ESP32 Case (Autodesk Fusion 360 design; units mm, degrees)
Autodesk Fusion 360 part; units mm, degrees
sketch "ESP32 Base" plane through (0, 0, 0) normal (0, 1, 0) x (1, 0, 0)
  line L0 (0, 0) -> (28, 0)
  line L1 (28, 0) -> (28, 55)
  line L2 (28, 55) -> (0, 55)
  line L3 (0, 55) -> (0, 0)
  line L4 (-2, 57) -> (30, 57)
  line L5 (30, 57) -> (30, -2)
  line L6 (30, -2) -> (-2, -2)
  line L7 (-2, -2) -> (-2, 57)
  dimension "d1" = 28
  dimension "d2" = 55
  dimension "d3" = 2
  dimension "d4" = 2
  dimension "d5" = 2
  dimension "d6" = 2
  constraint horizontal L0
  constraint vertical L1
  constraint horizontal L2
  constraint vertical L3
  constraint coincident L0.start L3.end
  constraint horizontal L4
  constraint vertical L5
  constraint horizontal L6
  constraint vertical L7
  measures "d1" distance of L0.start L0.end
  measures "d2" distance of L0.start L2.end
  measures "d3" distance of L1 L5
  measures "d4" distance of L0 L6
  measures "d5" distance of L3 L7
  measures "d6" distance of L2 L4
sketch "ESP32 Front" plane through (0, 0, 0) normal (0, 0, 1) x (1, 0, 0)
  line L0 (0, 0) -> (28, 0)
  line L1 (28, 0) -> (28, 10)
  line L2 (28, 10) -> (0, 10)
  line L3 (0, 10) -> (0, 0)
  line L4 (9.5, 0) -> (18.5, 0)
  line L5 (18.5, 0) -> (18.5, 5)
  line L6 (18.5, 5) -> (9.5, 5)
  line L7 (9.5, 5) -> (9.5, 0)
  line L8 (-2, 12) -> (30, 12)
  line L9 (30, 12) -> (30, -2)
  line L10 (30, -2) -> (-2, -2)
  line L11 (-2, -2) -> (-2, 12)
  dimension "d7" = 28
  dimension "d8" = 10
  dimension "d9" = 9
  dimension "d10" = 5
  dimension "d11" = 9.5
  dimension "d12" = 2
  dimension "d13" = 2
  dimension "d14" = 2
  dimension "d15" = 2
  constraint horizontal L0
  constraint vertical L1
  constraint horizontal L2
  constraint vertical L3
  constraint coincident L0.start L3.end
  constraint horizontal L4
  constraint vertical L5
  constraint horizontal L6
  constraint vertical L7
  constraint coincident L0 L4.start
  constraint horizontal L8
  constraint vertical L9
  constraint horizontal L10
  constraint vertical L11
  measures "d7" distance of L0.start L0.end
  measures "d8" distance of L0.start L2.end
  measures "d9" distance of L4.start L4.end
  measures "d10" distance of L4.start L6.end
  measures "d11" distance of L3 L7
  measures "d12" distance of L2 L8
  measures "d13" distance of L1 L9
  measures "d14" distance of L3 L11
  measures "d15" distance of L0 L10
extrude "Extrude1" add sketch "ESP32 Base" along normal blind 2 from surface at -2 contours L0 L1 L2 L3 | L4 L5 L6 L7 makes body 1
extrude "Extrude2" add sketch "ESP32 Base" along normal blind 10 bodies 1
extrude "Extrude3" cut sketch "ESP32 Front" along normal blind 3 contours L0 L4 L5 L6 L7 bodies 1
sketch "ESP32 Lid" plane through (0, 0, 0) normal (0, 1, 0) x (1, 0, 0)
  line L0 (0, 0) -> (28, 0)
  line L1 (28, 0) -> (28, 55)
  line L2 (28, 55) -> (0, 55)
  line L3 (0, 55) -> (0, 0)
  line L4 (-2, 57) -> (30, 57)
  line L5 (30, 57) -> (30, -2)
  line L6 (30, -2) -> (-2, -2)
  line L7 (-2, -2) -> (-2, 57)
  line L8 (1.5, 53.5) -> (26.5, 53.5)
  line L9 (26.5, 53.5) -> (26.5, 1.5)
  line L10 (26.5, 1.5) -> (1.5, 1.5)
  line L11 (1.5, 1.5) -> (1.5, 53.5)
  dimension "d23" = 55
  dimension "d24" = 28
  dimension "d25" = 2
  dimension "d26" = 2
  dimension "d27" = 2
  dimension "d28" = 2
  dimension "d29" = 1.5
  dimension "d30" = 1.5
  dimension "d31" = 1.5
  dimension "d32" = 1.5
  constraint horizontal L0
  constraint vertical L1
  constraint horizontal L2
  constraint vertical L3
  constraint coincident L0.start L3.end
  constraint horizontal L4
  constraint vertical L5
  constraint horizontal L6
  constraint vertical L7
  constraint horizontal L8
  constraint vertical L9
  constraint horizontal L10
  constraint vertical L11
  measures "d23" distance of L0.start L2.end
  measures "d24" distance of L0.start L0.end
  measures "d25" distance of L2 L4
  measures "d26" distance of L1 L5
  measures "d27" distance of L0 L6
  measures "d28" distance of L3 L7
  measures "d29" distance of L2 L8
  measures "d30" distance of L1 L9
  measures "d31" distance of L3 L11
  measures "d32" distance of L0 L10
extrude "Extrude4" add sketch "ESP32 Lid" along normal blind 2 separate body contours L0 L1 L2 L3 | L4 L5 L6 L7 | L8 L9 L10 L11 makes body 2
extrude "Extrude5" add sketch "ESP32 Lid" along normal blind 5 contours L0 L1 L2 L3 bodies 2
fillet "Fillet1" radius 1.5 4 edges at (-2, 4, 2) (-2, 4, -57) (30, 4, 2) (30, 4, -57) on bodies 1
fillet "Fillet2" radius 1 4 edges at (18.5, 2.5, 2) (18.5, 2.5, 0) (9.5, 2.5, 0) (9.5, 2.5, 2) on bodies 1
fillet "Fillet3" radius 1.5 4 edges at (-2, 1, 2) (30, 1, 2) (30, 1, -57) (-2, 1, -57) on bodies 2
move_body "Move1" bodies 2 to x (1, 0, 0) y (0, 1, 0) z (0, 0, 1) at (45, 0, 0)
sketch "HomeAssistant" plane through (0, 0, 0) normal (0, 1, 0) x (1, 0, 0)
  spline S0 degree 3 poles (63.1801, 32.2819) (63.2605, 32.4605) (63.314, 32.6569) (63.314, 32.8623) knots 0 0 0 0 1 1 1 1
  spline S1 degree 3 poles (63.314, 32.8623) (63.314, 33.6035) (62.7157, 34.2018) (61.9746, 34.2018) knots 0 0 0 0 1 1 1 1
  spline S2 degree 3 poles (61.9746, 34.2018) (61.2334, 34.2018) (60.6351, 33.6035) (60.6351, 32.8623) knots 0 0 0 0 1 1 1 1
  spline S3 degree 3 poles (60.6351, 32.8623) (60.6351, 32.1211) (61.2334, 31.5229) (61.9746, 31.5229) knots 0 0 0 0 1 1 1 1
  spline S4 degree 3 poles (61.9746, 31.5229) (62.18, 31.5229) (62.3764, 31.5675) (62.555, 31.6568) knots 0 0 0 0 1 1 1 1
  line L0 (62.555, 31.6568) -> (64.4749, 29.728)
  line L1 (64.4749, 29.728) -> (64.4749, 27.8617)
  line L2 (64.4749, 27.8617) -> (62.0639, 25.4417)
  line L3 (62.0639, 25.4417) -> (62.0639, 27.2098)
  spline S5 degree 3 poles (62.0639, 27.2098) (62.5818, 27.3973) (62.9569, 27.8885) (62.9569, 28.4778) knots 0 0 0 0 1 1 1 1
  spline S6 degree 3 poles (62.9569, 28.4778) (62.9569, 29.219) (62.3586, 29.8173) (61.6174, 29.8173) knots 0 0 0 0 1 1 1 1
  spline S7 degree 3 poles (61.6174, 29.8173) (60.8762, 29.8173) (60.2779, 29.219) (60.2779, 28.4778) knots 0 0 0 0 1 1 1 1
  spline S8 degree 3 poles (60.2779, 28.4778) (60.2779, 27.8974) (60.653, 27.3973) (61.1709, 27.2098) knots 0 0 0 0 1 1 1 1
  line L4 (61.1709, 27.2098) -> (61.1709, 24.5398)
  line L5 (61.1709, 24.5398) -> (58.9385, 22.2985)
  line L6 (58.9385, 22.2985) -> (58.9385, 35.4519)
  line L7 (58.9385, 35.4519) -> (60.7691, 37.2914)
  spline S9 degree 3 poles (60.7691, 37.2914) (60.9477, 37.2111) (61.1352, 37.1575) (61.3495, 37.1575) knots 0 0 0 0 1 1 1 1
  spline S10 degree 3 poles (61.3495, 37.1575) (62.0907, 37.1575) (62.689, 37.7558) (62.689, 38.4969) knots 0 0 0 0 1 1 1 1
  spline S11 degree 3 poles (62.689, 38.4969) (62.689, 39.2381) (62.0907, 39.8364) (61.3495, 39.8364) knots 0 0 0 0 1 1 1 1
  spline S12 degree 3 poles (61.3495, 39.8364) (60.6083, 39.8364) (60.0101, 39.2381) (60.0101, 38.4969) knots 0 0 0 0 1 1 1 1
  spline S13 degree 3 poles (60.0101, 38.4969) (60.0101, 38.2916) (60.0547, 38.0951) (60.144, 37.9165) knots 0 0 0 0 1 1 1 1
  line L8 (60.144, 37.9165) -> (58.5009, 36.2645)
  line L9 (58.5009, 36.2645) -> (56.8579, 37.9165)
  spline S14 degree 3 poles (56.8579, 37.9165) (56.9382, 38.0951) (56.9918, 38.2916) (56.9918, 38.4969) knots 0 0 0 0 1 1 1 1
  spline S15 degree 3 poles (56.9918, 38.4969) (56.9918, 39.2381) (56.3935, 39.8364) (55.6524, 39.8364) knots 0 0 0 0 1 1 1 1
  spline S16 degree 3 poles (55.6524, 39.8364) (54.9112, 39.8364) (54.3129, 39.2381) (54.3129, 38.4969) knots 0 0 0 0 1 1 1 1
  spline S17 degree 3 poles (54.3129, 38.4969) (54.3129, 37.7558) (54.9112, 37.1575) (55.6524, 37.1575) knots 0 0 0 0 1 1 1 1
  spline S18 degree 3 poles (55.6524, 37.1575) (55.8577, 37.1575) (56.0542, 37.2021) (56.2328, 37.2914) knots 0 0 0 0 1 1 1 1
  line L10 (56.2328, 37.2914) -> (58.0634, 35.4519)
  line L11 (58.0634, 35.4519) -> (58.0634, 26.0579)
  line L12 (58.0634, 26.0579) -> (54.8487, 29.2815)
  line L13 (54.8487, 29.2815) -> (54.8487, 31.8622)
  spline S19 degree 3 poles (54.8487, 31.8622) (55.3666, 32.0497) (55.7417, 32.5408) (55.7417, 33.1302) knots 0 0 0 0 1 1 1 1
  spline S20 degree 3 poles (55.7417, 33.1302) (55.7417, 33.8714) (55.1434, 34.4696) (54.4022, 34.4696) knots 0 0 0 0 1 1 1 1
  spline S21 degree 3 poles (54.4022, 34.4696) (53.661, 34.4696) (53.0628, 33.8714) (53.0628, 33.1302) knots 0 0 0 0 1 1 1 1
  spline S22 degree 3 poles (53.0628, 33.1302) (53.0628, 32.5498) (53.4378, 32.0497) (53.9557, 31.8622) knots 0 0 0 0 1 1 1 1
  line L14 (53.9557, 31.8622) -> (53.9557, 30.1834)
  line L15 (53.9557, 30.1834) -> (51.4554, 32.6926)
  line L16 (51.4554, 32.6926) -> (51.4554, 35.184)
  spline S23 degree 3 poles (51.4554, 35.184) (51.9733, 35.3715) (52.3484, 35.8627) (52.3484, 36.452) knots 0 0 0 0 1 1 1 1
  spline S24 degree 3 poles (52.3484, 36.452) (52.3484, 37.1932) (51.7501, 37.7915) (51.0089, 37.7915) knots 0 0 0 0 1 1 1 1
  spline S25 degree 3 poles (51.0089, 37.7915) (50.2678, 37.7915) (49.6695, 37.1932) (49.6695, 36.452) knots 0 0 0 0 1 1 1 1
  spline S26 degree 3 poles (49.6695, 36.452) (49.6695, 35.8716) (50.0445, 35.3715) (50.5624, 35.184) knots 0 0 0 0 1 1 1 1
  line L17 (50.5624, 35.184) -> (50.5624, 32.3265)
  line L18 (50.5624, 32.3265) -> (53.3217, 29.5583)
  line L19 (53.3217, 29.5583) -> (51.7233, 29.5583)
  spline S27 degree 3 poles (51.7233, 29.5583) (51.5358, 30.0762) (51.0446, 30.4513) (50.4642, 30.4513) knots 0 0 0 0 1 1 1 1
  spline S28 degree 3 poles (50.4642, 30.4513) (49.7231, 30.4513) (49.1248, 29.853) (49.1248, 29.1118) knots 0 0 0 0 1 1 1 1
  spline S29 degree 3 poles (49.1248, 29.1118) (49.1248, 28.3707) (49.7231, 27.7724) (50.4642, 27.7724) knots 0 0 0 0 1 1 1 1
  spline S30 degree 3 poles (50.4642, 27.7724) (51.0446, 27.7724) (51.5447, 28.1474) (51.7233, 28.6654) knots 0 0 0 0 1 1 1 1
  line L20 (51.7233, 28.6654) -> (54.2058, 28.6654)
  line L21 (54.2058, 28.6654) -> (58.0455, 24.8077)
  line L22 (58.0455, 24.8077) -> (58.0455, 18.1015)
  line L23 (58.0455, 18.1015) -> (55.9917, 20.1643)
  line L24 (55.9917, 20.1643) -> (55.9917, 22.745)
  spline S31 degree 3 poles (55.9917, 22.745) (56.5096, 22.9325) (56.8847, 23.4236) (56.8847, 24.013) knots 0 0 0 0 1 1 1 1
  spline S32 degree 3 poles (56.8847, 24.013) (56.8847, 24.7541) (56.2864, 25.3524) (55.5452, 25.3524) knots 0 0 0 0 1 1 1 1
  spline S33 degree 3 poles (55.5452, 25.3524) (54.804, 25.3524) (54.2058, 24.7541) (54.2058, 24.013) knots 0 0 0 0 1 1 1 1
  spline S34 degree 3 poles (54.2058, 24.013) (54.2058, 23.4326) (54.5808, 22.9325) (55.0987, 22.745) knots 0 0 0 0 1 1 1 1
  line L25 (55.0987, 22.745) -> (55.0987, 21.0662)
  line L26 (55.0987, 21.0662) -> (52.1162, 24.0666)
  spline S35 degree 3 poles (52.1162, 24.0666) (52.1966, 24.2452) (52.2502, 24.4416) (52.2502, 24.647) knots 0 0 0 0 1 1 1 1
  spline S36 degree 3 poles (52.2502, 24.647) (52.2502, 25.3882) (51.6519, 25.9864) (50.9107, 25.9864) knots 0 0 0 0 1 1 1 1
  spline S37 degree 3 poles (50.9107, 25.9864) (50.1695, 25.9864) (49.5712, 25.3882) (49.5712, 24.647) knots 0 0 0 0 1 1 1 1
  spline S38 degree 3 poles (49.5712, 24.647) (49.5712, 23.9058) (50.1695, 23.3075) (50.9107, 23.3075) knots 0 0 0 0 1 1 1 1
  spline S39 degree 3 poles (50.9107, 23.3075) (51.1161, 23.3075) (51.3125, 23.3522) (51.4911, 23.4415) knots 0 0 0 0 1 1 1 1
  line L27 (51.4911, 23.4415) -> (54.4736, 20.4411)
  line L28 (54.4736, 20.4411) -> (52.8842, 20.4411)
  spline S40 degree 3 poles (52.8842, 20.4411) (52.6966, 20.959) (52.2055, 21.3341) (51.6251, 21.3341) knots 0 0 0 0 1 1 1 1
  spline S41 degree 3 poles (51.6251, 21.3341) (50.8839, 21.3341) (50.2856, 20.7358) (50.2856, 19.9946) knots 0 0 0 0 1 1 1 1
  spline S42 degree 3 poles (50.2856, 19.9946) (50.2856, 19.2535) (50.8839, 18.6552) (51.6251, 18.6552) knots 0 0 0 0 1 1 1 1
  spline S43 degree 3 poles (51.6251, 18.6552) (52.2055, 18.6552) (52.7056, 19.0302) (52.8842, 19.5481) knots 0 0 0 0 1 1 1 1
  line L29 (52.8842, 19.5481) -> (55.3666, 19.5481)
  line L30 (55.3666, 19.5481) -> (57.8669, 17.0389)
  line L31 (57.8669, 17.0389) -> (59.126, 17.0389)
  line L32 (59.126, 17.0389) -> (61.7156, 19.6374)
  line L33 (61.7156, 19.6374) -> (64.1088, 19.6374)
  spline S44 degree 3 poles (64.1088, 19.6374) (64.2963, 19.1195) (64.7874, 18.7445) (65.3679, 18.7445) knots 0 0 0 0 1 1 1 1
  spline S45 degree 3 poles (65.3679, 18.7445) (66.109, 18.7445) (66.7073, 19.3428) (66.7073, 20.0839) knots 0 0 0 0 1 1 1 1
  spline S46 degree 3 poles (66.7073, 20.0839) (66.7073, 20.8251) (66.109, 21.4234) (65.3679, 21.4234) knots 0 0 0 0 1 1 1 1
  spline S47 degree 3 poles (65.3679, 21.4234) (64.7874, 21.4234) (64.2874, 21.0483) (64.1088, 20.5304) knots 0 0 0 0 1 1 1 1
  line L34 (64.1088, 20.5304) -> (61.3495, 20.5304)
  line L35 (61.3495, 20.5304) -> (58.9474, 18.1194)
  line L36 (58.9474, 18.1194) -> (58.9474, 21.0662)
  line L37 (58.9474, 21.0662) -> (61.8049, 23.9415)
  line L38 (61.8049, 23.9415) -> (66.4216, 23.9415)
  spline S48 degree 3 poles (66.4216, 23.9415) (66.6091, 23.4236) (67.1002, 23.0486) (67.6807, 23.0486) knots 0 0 0 0 1 1 1 1
  spline S49 degree 3 poles (67.6807, 23.0486) (68.4218, 23.0486) (69.0201, 23.6469) (69.0201, 24.388) knots 0 0 0 0 1 1 1 1
  spline S50 degree 3 poles (69.0201, 24.388) (69.0201, 25.1292) (68.4218, 25.7275) (67.6807, 25.7275) knots 0 0 0 0 1 1 1 1
  spline S51 degree 3 poles (67.6807, 25.7275) (67.1002, 25.7275) (66.6002, 25.3524) (66.4216, 24.8345) knots 0 0 0 0 1 1 1 1
  line L39 (66.4216, 24.8345) -> (62.6979, 24.8345)
  line L40 (62.6979, 24.8345) -> (65.3679, 27.5134)
  line L41 (65.3679, 27.5134) -> (65.3679, 29.7548)
  line L42 (65.3679, 29.7548) -> (67.2877, 31.6836)
  spline S52 degree 3 poles (67.2877, 31.6836) (67.4663, 31.6032) (67.6539, 31.5496) (67.8682, 31.5496) knots 0 0 0 0 1 1 1 1
  spline S53 degree 3 poles (67.8682, 31.5496) (68.6093, 31.5496) (69.2076, 32.1479) (69.2076, 32.8891) knots 0 0 0 0 1 1 1 1
  spline S54 degree 3 poles (69.2076, 32.8891) (69.2076, 33.6303) (68.6093, 34.2285) (67.8682, 34.2285) knots 0 0 0 0 1 1 1 1
  spline S55 degree 3 poles (67.8682, 34.2285) (67.127, 34.2285) (66.5287, 33.6303) (66.5287, 32.8891) knots 0 0 0 0 1 1 1 1
  spline S56 degree 3 poles (66.5287, 32.8891) (66.5287, 32.6837) (66.5734, 32.4873) (66.6627, 32.3087) knots 0 0 0 0 1 1 1 1
  line L43 (66.6627, 32.3087) -> (65.3679, 31.0139)
  line L44 (65.3679, 31.0139) -> (65.3679, 35.1126)
  spline S57 degree 3 poles (65.3679, 35.1126) (65.8858, 35.3001) (66.2608, 35.7912) (66.2608, 36.3806) knots 0 0 0 0 1 1 1 1
  spline S58 degree 3 poles (66.2608, 36.3806) (66.2608, 37.1218) (65.6625, 37.7201) (64.9214, 37.7201) knots 0 0 0 0 1 1 1 1
  spline S59 degree 3 poles (64.9214, 37.7201) (64.1802, 37.7201) (63.5819, 37.1218) (63.5819, 36.3806) knots 0 0 0 0 1 1 1 1
  spline S60 degree 3 poles (63.5819, 36.3806) (63.5819, 35.8002) (63.957, 35.3001) (64.4749, 35.1126) knots 0 0 0 0 1 1 1 1
  line L45 (64.4749, 35.1126) -> (64.4749, 31.0139)
  line L46 (64.4749, 31.0139) -> (63.1801, 32.2819)
sketch "Sketch6" plane through (0, 0, 0) normal (0, 1, 0) x (1, 0, 0)
  line L0 (36.9451, 52.3701) -> (79.5148, 52.3701)
  line L1 (79.5148, 52.3701) -> (79.5148, 14.6379)
  line L2 (79.5148, 14.6379) -> (36.9451, 14.6379)
  line L3 (36.9451, 14.6379) -> (36.9451, 52.3701)
  spline S0 degree 3 poles (63.8629, 33.0203) (63.9596, 33.2353) (64.0241, 33.4718) (64.0241, 33.719) knots 0 0 0 0 1 1 1 1
  spline S1 degree 3 poles (64.0241, 33.719) (64.0241, 34.6113) (63.3039, 35.3315) (62.4116, 35.3315) knots 0 0 0 0 1 1 1 1
  spline S2 degree 3 poles (62.4116, 35.3315) (61.5194, 35.3315) (60.7992, 34.6113) (60.7992, 33.719) knots 0 0 0 0 1 1 1 1
  spline S3 degree 3 poles (60.7992, 33.719) (60.7992, 32.8268) (61.5194, 32.1065) (62.4116, 32.1065) knots 0 0 0 0 1 1 1 1
  spline S4 degree 3 poles (62.4116, 32.1065) (62.6589, 32.1065) (62.8954, 32.1603) (63.1104, 32.2678) knots 0 0 0 0 1 1 1 1
  line L4 (63.1104, 32.2678) -> (65.4216, 29.9458)
  line L5 (65.4216, 29.9458) -> (65.4216, 27.6991)
  line L6 (65.4216, 27.6991) -> (62.5191, 24.7859)
  line L7 (62.5191, 24.7859) -> (62.5191, 26.9143)
  spline S5 degree 3 poles (62.5191, 26.9143) (63.1426, 27.1401) (63.5941, 27.7313) (63.5941, 28.4408) knots 0 0 0 0 1 1 1 1
  spline S6 degree 3 poles (63.5941, 28.4408) (63.5941, 29.3331) (62.8739, 30.0533) (61.9816, 30.0533) knots 0 0 0 0 1 1 1 1
  spline S7 degree 3 poles (61.9816, 30.0533) (61.0894, 30.0533) (60.3692, 29.3331) (60.3692, 28.4408) knots 0 0 0 0 1 1 1 1
  spline S8 degree 3 poles (60.3692, 28.4408) (60.3692, 27.7421) (60.8207, 27.1401) (61.4442, 26.9143) knots 0 0 0 0 1 1 1 1
  line L8 (61.4442, 26.9143) -> (61.4442, 23.7001)
  line L9 (61.4442, 23.7001) -> (58.7567, 21.0019)
  line L10 (58.7567, 21.0019) -> (58.7567, 36.8365)
  line L11 (58.7567, 36.8365) -> (60.9604, 39.051)
  spline S9 degree 3 poles (60.9604, 39.051) (61.1754, 38.9542) (61.4012, 38.8897) (61.6592, 38.8897) knots 0 0 0 0 1 1 1 1
  spline S10 degree 3 poles (61.6592, 38.8897) (62.5514, 38.8897) (63.2716, 39.61) (63.2716, 40.5022) knots 0 0 0 0 1 1 1 1
  spline S11 degree 3 poles (63.2716, 40.5022) (63.2716, 41.3945) (62.5514, 42.1147) (61.6592, 42.1147) knots 0 0 0 0 1 1 1 1
  spline S12 degree 3 poles (61.6592, 42.1147) (60.7669, 42.1147) (60.0467, 41.3945) (60.0467, 40.5022) knots 0 0 0 0 1 1 1 1
  spline S13 degree 3 poles (60.0467, 40.5022) (60.0467, 40.255) (60.1004, 40.0185) (60.2079, 39.8035) knots 0 0 0 0 1 1 1 1
  line L12 (60.2079, 39.8035) -> (58.2299, 37.8148)
  line L13 (58.2299, 37.8148) -> (56.2519, 39.8035)
  spline S14 degree 3 poles (56.2519, 39.8035) (56.3487, 40.0185) (56.4132, 40.255) (56.4132, 40.5022) knots 0 0 0 0 1 1 1 1
  spline S15 degree 3 poles (56.4132, 40.5022) (56.4132, 41.3945) (55.6929, 42.1147) (54.8007, 42.1147) knots 0 0 0 0 1 1 1 1
  spline S16 degree 3 poles (54.8007, 42.1147) (53.9085, 42.1147) (53.1882, 41.3945) (53.1882, 40.5022) knots 0 0 0 0 1 1 1 1
  spline S17 degree 3 poles (53.1882, 40.5022) (53.1882, 39.61) (53.9085, 38.8897) (54.8007, 38.8897) knots 0 0 0 0 1 1 1 1
  spline S18 degree 3 poles (54.8007, 38.8897) (55.048, 38.8897) (55.2845, 38.9435) (55.4995, 39.051) knots 0 0 0 0 1 1 1 1
  line L14 (55.4995, 39.051) -> (57.7032, 36.8365)
  line L15 (57.7032, 36.8365) -> (57.7032, 25.5276)
  line L16 (57.7032, 25.5276) -> (53.8332, 29.4083)
  line L17 (53.8332, 29.4083) -> (53.8332, 32.515)
  spline S19 degree 3 poles (53.8332, 32.515) (54.4567, 32.7408) (54.9082, 33.332) (54.9082, 34.0415) knots 0 0 0 0 1 1 1 1
  spline S20 degree 3 poles (54.9082, 34.0415) (54.9082, 34.9338) (54.188, 35.654) (53.2957, 35.654) knots 0 0 0 0 1 1 1 1
  spline S21 degree 3 poles (53.2957, 35.654) (52.4035, 35.654) (51.6832, 34.9338) (51.6832, 34.0415) knots 0 0 0 0 1 1 1 1
  spline S22 degree 3 poles (51.6832, 34.0415) (51.6832, 33.3428) (52.1347, 32.7408) (52.7582, 32.515) knots 0 0 0 0 1 1 1 1
  line L18 (52.7582, 32.515) -> (52.7582, 30.4941)
  line L19 (52.7582, 30.4941) -> (49.7482, 33.5148)
  line L20 (49.7482, 33.5148) -> (49.7482, 36.514)
  spline S23 degree 3 poles (49.7482, 36.514) (50.3717, 36.7398) (50.8232, 37.331) (50.8232, 38.0405) knots 0 0 0 0 1 1 1 1
  spline S24 degree 3 poles (50.8232, 38.0405) (50.8232, 38.9327) (50.103, 39.653) (49.2107, 39.653) knots 0 0 0 0 1 1 1 1
  spline S25 degree 3 poles (49.2107, 39.653) (48.3185, 39.653) (47.5983, 38.9327) (47.5983, 38.0405) knots 0 0 0 0 1 1 1 1
  spline S26 degree 3 poles (47.5983, 38.0405) (47.5983, 37.3418) (48.0498, 36.7398) (48.6733, 36.514) knots 0 0 0 0 1 1 1 1
  line L21 (48.6733, 36.514) -> (48.6733, 33.074)
  line L22 (48.6733, 33.074) -> (51.995, 29.7416)
  line L23 (51.995, 29.7416) -> (50.0707, 29.7416)
  spline S27 degree 3 poles (50.0707, 29.7416) (49.845, 30.3651) (49.2537, 30.8166) (48.555, 30.8166) knots 0 0 0 0 1 1 1 1
  spline S28 degree 3 poles (48.555, 30.8166) (47.6628, 30.8166) (46.9425, 30.0963) (46.9425, 29.2041) knots 0 0 0 0 1 1 1 1
  spline S29 degree 3 poles (46.9425, 29.2041) (46.9425, 28.3118) (47.6628, 27.5916) (48.555, 27.5916) knots 0 0 0 0 1 1 1 1
  spline S30 degree 3 poles (48.555, 27.5916) (49.2537, 27.5916) (49.8557, 28.0431) (50.0707, 28.6666) knots 0 0 0 0 1 1 1 1
  line L24 (50.0707, 28.6666) -> (53.0592, 28.6666)
  line L25 (53.0592, 28.6666) -> (57.6817, 24.0226)
  line L26 (57.6817, 24.0226) -> (57.6817, 15.9494)
  line L27 (57.6817, 15.9494) -> (55.2092, 18.4327)
  line L28 (55.2092, 18.4327) -> (55.2092, 21.5394)
  spline S31 degree 3 poles (55.2092, 21.5394) (55.8327, 21.7651) (56.2842, 22.3564) (56.2842, 23.0659) knots 0 0 0 0 1 1 1 1
  spline S32 degree 3 poles (56.2842, 23.0659) (56.2842, 23.9581) (55.5639, 24.6784) (54.6717, 24.6784) knots 0 0 0 0 1 1 1 1
  spline S33 degree 3 poles (54.6717, 24.6784) (53.7795, 24.6784) (53.0592, 23.9581) (53.0592, 23.0659) knots 0 0 0 0 1 1 1 1
  spline S34 degree 3 poles (53.0592, 23.0659) (53.0592, 22.3671) (53.5107, 21.7651) (54.1342, 21.5394) knots 0 0 0 0 1 1 1 1
  line L29 (54.1342, 21.5394) -> (54.1342, 19.5184)
  line L30 (54.1342, 19.5184) -> (50.5437, 23.1304)
  spline S35 degree 3 poles (50.5437, 23.1304) (50.6405, 23.3454) (50.705, 23.5819) (50.705, 23.8291) knots 0 0 0 0 1 1 1 1
  spline S36 degree 3 poles (50.705, 23.8291) (50.705, 24.7214) (49.9847, 25.4416) (49.0925, 25.4416) knots 0 0 0 0 1 1 1 1
  spline S37 degree 3 poles (49.0925, 25.4416) (48.2003, 25.4416) (47.48, 24.7214) (47.48, 23.8291) knots 0 0 0 0 1 1 1 1
  spline S38 degree 3 poles (47.48, 23.8291) (47.48, 22.9369) (48.2003, 22.2166) (49.0925, 22.2166) knots 0 0 0 0 1 1 1 1
  spline S39 degree 3 poles (49.0925, 22.2166) (49.3397, 22.2166) (49.5762, 22.2704) (49.7912, 22.3779) knots 0 0 0 0 1 1 1 1
  line L31 (49.7912, 22.3779) -> (53.3817, 18.7659)
  line L32 (53.3817, 18.7659) -> (51.4682, 18.7659)
  spline S40 degree 3 poles (51.4682, 18.7659) (51.2425, 19.3894) (50.6512, 19.8409) (49.9525, 19.8409) knots 0 0 0 0 1 1 1 1
  spline S41 degree 3 poles (49.9525, 19.8409) (49.0603, 19.8409) (48.34, 19.1207) (48.34, 18.2284) knots 0 0 0 0 1 1 1 1
  spline S42 degree 3 poles (48.34, 18.2284) (48.34, 17.3362) (49.0603, 16.6159) (49.9525, 16.6159) knots 0 0 0 0 1 1 1 1
  spline S43 degree 3 poles (49.9525, 16.6159) (50.6512, 16.6159) (51.2532, 17.0674) (51.4682, 17.6909) knots 0 0 0 0 1 1 1 1
  line L33 (51.4682, 17.6909) -> (54.4567, 17.6909)
  line L34 (54.4567, 17.6909) -> (57.4667, 14.6702)
  line L35 (57.4667, 14.6702) -> (58.9824, 14.6702)
  line L36 (58.9824, 14.6702) -> (62.0999, 17.7984)
  line L37 (62.0999, 17.7984) -> (64.9809, 17.7984)
  spline S44 degree 3 poles (64.9809, 17.7984) (65.2066, 17.1749) (65.7979, 16.7234) (66.4966, 16.7234) knots 0 0 0 0 1 1 1 1
  spline S45 degree 3 poles (66.4966, 16.7234) (67.3889, 16.7234) (68.1091, 17.4437) (68.1091, 18.3359) knots 0 0 0 0 1 1 1 1
  spline S46 degree 3 poles (68.1091, 18.3359) (68.1091, 19.2281) (67.3889, 19.9484) (66.4966, 19.9484) knots 0 0 0 0 1 1 1 1
  spline S47 degree 3 poles (66.4966, 19.9484) (65.7979, 19.9484) (65.1959, 19.4969) (64.9809, 18.8734) knots 0 0 0 0 1 1 1 1
  line L38 (64.9809, 18.8734) -> (61.6592, 18.8734)
  line L39 (61.6592, 18.8734) -> (58.7674, 15.9709)
  line L40 (58.7674, 15.9709) -> (58.7674, 19.5184)
  line L41 (58.7674, 19.5184) -> (62.2074, 22.9799)
  line L42 (62.2074, 22.9799) -> (67.7651, 22.9799)
  spline S48 degree 3 poles (67.7651, 22.9799) (67.9909, 22.3564) (68.5821, 21.9049) (69.2808, 21.9049) knots 0 0 0 0 1 1 1 1
  spline S49 degree 3 poles (69.2808, 21.9049) (70.1731, 21.9049) (70.8933, 22.6251) (70.8933, 23.5174) knots 0 0 0 0 1 1 1 1
  spline S50 degree 3 poles (70.8933, 23.5174) (70.8933, 24.4096) (70.1731, 25.1299) (69.2808, 25.1299) knots 0 0 0 0 1 1 1 1
  spline S51 degree 3 poles (69.2808, 25.1299) (68.5821, 25.1299) (67.9801, 24.6784) (67.7651, 24.0549) knots 0 0 0 0 1 1 1 1
  line L43 (67.7651, 24.0549) -> (63.2824, 24.0549)
  line L44 (63.2824, 24.0549) -> (66.4966, 27.2798)
  line L45 (66.4966, 27.2798) -> (66.4966, 29.9781)
  line L46 (66.4966, 29.9781) -> (68.8078, 32.3001)
  spline S52 degree 3 poles (68.8078, 32.3001) (69.0228, 32.2033) (69.2486, 32.1388) (69.5066, 32.1388) knots 0 0 0 0 1 1 1 1
  spline S53 degree 3 poles (69.5066, 32.1388) (70.3988, 32.1388) (71.1191, 32.859) (71.1191, 33.7513) knots 0 0 0 0 1 1 1 1
  spline S54 degree 3 poles (71.1191, 33.7513) (71.1191, 34.6435) (70.3988, 35.3638) (69.5066, 35.3638) knots 0 0 0 0 1 1 1 1
  spline S55 degree 3 poles (69.5066, 35.3638) (68.6143, 35.3638) (67.8941, 34.6435) (67.8941, 33.7513) knots 0 0 0 0 1 1 1 1
  spline S56 degree 3 poles (67.8941, 33.7513) (67.8941, 33.504) (67.9479, 33.2675) (68.0554, 33.0525) knots 0 0 0 0 1 1 1 1
  line L47 (68.0554, 33.0525) -> (66.4966, 31.4938)
  line L48 (66.4966, 31.4938) -> (66.4966, 36.428)
  spline S57 degree 3 poles (66.4966, 36.428) (67.1201, 36.6538) (67.5716, 37.245) (67.5716, 37.9545) knots 0 0 0 0 1 1 1 1
  spline S58 degree 3 poles (67.5716, 37.9545) (67.5716, 38.8467) (66.8514, 39.567) (65.9591, 39.567) knots 0 0 0 0 1 1 1 1
  spline S59 degree 3 poles (65.9591, 39.567) (65.0669, 39.567) (64.3466, 38.8467) (64.3466, 37.9545) knots 0 0 0 0 1 1 1 1
  spline S60 degree 3 poles (64.3466, 37.9545) (64.3466, 37.2558) (64.7981, 36.6538) (65.4216, 36.428) knots 0 0 0 0 1 1 1 1
  line L49 (65.4216, 36.428) -> (65.4216, 31.4938)
  line L50 (65.4216, 31.4938) -> (63.8629, 33.0203)
extrude "Extrude7" cut sketch "Sketch6" along normal blind 10 from surface at -2 contours S0 S1 S2 S3 S4 L4 L5 L6 L7 S5 S6 S7 S8 L8 L9 L10 L11 S9 S10 S11 S12 S13 L12 L13 S14 S15 S16 S17 S18 L14 L15 L16 L17 S19 S20 S21 S22 L18 L19 L20 S23 S24 S25 S26 L21 L22 L23 S27 S28 S29 S30 L24 L25 L26 L27 L28 S31 S32 S33 S34 L29 L30 S35 S36 S37 S38 S39 L31 L32 S40 S41 S42 S43 L33 L34 L35 L36 L37 S44 S45 S46 S47 L38 L39 L40 L41 L42 S48 S49 S50 S51 L43 L44 L45 L46 S52 S53 S54 S55 S56 L47 L48 S57 S58 S59 S60 L49 L50 bodies 2
named bodies: "Case", "Lid"
